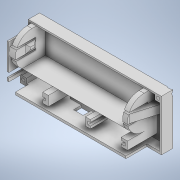
# Autodesk Inventor part: batteryholder18650
Saved by Autodesk Inventor 2022 (Build 260153000, 153)
## iProperties
Created: 2021-01-11
Part Number: batteryholder18650
Material: Generic
Document SubType Name: Modeling
Designer: papa
Density: 1 g/cm^3
Appearance: Default
Author: papa
Autodesk Inventor part; units mm, degrees
ref_plane "YZ Plane" through (0, 0, 0) normal (1, 0, 0) x (0, 1, 0)
ref_plane "XZ Plane" through (0, 0, 0) normal (0, 1, 0) x (-1, 0, 0)
ref_plane "XY Plane" through (0, 0, 0) normal (0, 0, 1) x (1, 0, 0)
sketch "Sketch1" plane through (0, 0, 0) normal (0, 0, 1) x (1, 0, 0)
  line L0 (0, 0) -> (82.5, 0)
  line L1 (82.5, 0) -> (82.5, 31.5)
  line L2 (82.5, 31.5) -> (0, 31.5)
  line L3 (0, 31.5) -> (0, 0)
  line L4 (1, 30.5) -> (81.5, 30.5)
  line L5 (81.5, 30.5) -> (81.5, 1.5)
  line L6 (81.5, 1.5) -> (1, 1.5)
  line L7 (1, 1.5) -> (1, 30.5)
  line L8 (81.5, 30.5) -> (78.5, 30.5)
  line L9 (78.5, 30.5) -> (78.5, 27.5)
  line L10 (78.5, 27.5) -> (81.5, 27.5)
  line L11 (81.5, 27.5) -> (81.5, 30.5)
  line L12 (1, 1.5) -> (4, 1.5)
  line L13 (4, 1.5) -> (4, 4.5)
  line L14 (4, 4.5) -> (1, 4.5)
  line L15 (1, 4.5) -> (1, 1.5)
  point P0 (78.5, 30.5)
  point P1 (1, 4.5)
  dimension "d0" = 82.5
  dimension "d1" = 31.5
  dimension "d2" = 1
  dimension "d3" = 1
  dimension "d4" = 1.5
  dimension "d5" = 1
  dimension "d26" = 4
  dimension "d27" = 4.5
  dimension "d28" = 4
  dimension "d29" = 4
  constraints: 32 end point, 8 parallel, 4 horizontal, 4 perpendicular
  measures "d0" distance of L2.end L1.end
  measures "d1" distance of L1.end L0.end
  measures "d2" distance between parallel lines of L4 L2
  measures "d3" distance between parallel lines of L3 L7
  measures "d4" distance between parallel lines of L0 L6
  measures "d5" distance between parallel lines of L1 L5
  measures "d26" distance between parallel lines of L3 L13
  measures "d27" distance between parallel lines of L0 L14
  measures "d28" distance between parallel lines of L2 L10
  measures "d29" distance between parallel lines of L1 L9
extrude "Extrusion1" add sketch "Sketch1" along normal blind 1.5 contours L3 L2 L1 L0 | L4 L9 L10 L5 L6 L13 L14 L7 | L4 L5 L10 L9 | L14 L13 L6 L7
extrude "Extrusion2" add sketch "Sketch1" along normal blind 20 contours L3 L2 L1 L0 | L4 L5 L10 L9 | L14 L13 L6 L7
sketch "Sketch2" plane through (0, 0, 0) normal (0, 0, -1) x (-1, 0, 0)
  circle A0 centre (-2, 2.5) radius 1
  circle A1 centre (-80.5, 29.5) radius 1
  line L0 (0, 0) -> (-82.5, 0) projected
  line L1 (0, 31.5) -> (0, 0) projected
  line L2 (-82.5, 0) -> (-82.5, 31.5) projected
  line L3 (-82.5, 31.5) -> (0, 31.5) projected
  dimension "d10" = 2
  dimension "d11" = 2
  dimension "d12" = 2.5
  dimension "d13" = 2
  dimension "d14" = 2
  dimension "d15" = 2
  constraints: 2 centre point
  measures "d10" diameter of A0
  measures "d11" diameter of A1
  measures "d12" distance from line of L0 A0.centre
  measures "d13" distance from line of L1 A0.centre
  measures "d14" distance from line of L2 A1.centre
  measures "d15" distance from line of L3 A1.centre
extrude "Extrusion3" cut sketch "Sketch2" against normal through all contours A0 | A1
sketch "Sketch3" plane through (0, 0, 20) normal (0, 0, 1) x (1, 0, 0)
  line L0 (82.5, 0) -> (82.5, 31.5) projected
  line L1 (0, 31.5) -> (82.5, 31.5)
  line L2 (82.5, 31.5) -> (82.5, 26.5)
  line L3 (82.5, 26.5) -> (0, 26.5)
  line L4 (0, 26.5) -> (0, 31.5)
  line L5 (0, 0) -> (5, 0)
  line L6 (5, 0) -> (5, 5)
  line L7 (5, 5) -> (0, 5)
  line L8 (0, 5) -> (0, 0)
  line L9 (82.5, 31.5) -> (0, 31.5) projected
  line L10 (82.5, 0) -> (73.5, 0)
  line L11 (73.5, 0) -> (73.5, 26.5)
  line L12 (73.5, 26.5) -> (82.5, 26.5)
  line L13 (82.5, 26.5) -> (82.5, 0)
  point P0 (1, 1.5)
  dimension "d20" = 5
  dimension "d21" = 5
  dimension "d22" = 5
  dimension "d125" = 9
  constraints: 24 end point, 6 parallel, 3 collinear, 3 horizontal, 3 perpendicular, 1 point on line
  measures "d20" distance between parallel lines of L1 L3
  measures "d21" distance between parallel lines of L8 L6
  measures "d22" distance of L7.end L5.start
  measures "d125" distance between parallel lines of L0 L11
extrude "Extrusion4" cut sketch "Sketch3" against normal blind 8
thicken "Thicken1" operation add thickness 5 both sides no extend neighbours yes toward (0, 0, -1) faces at (27.8333, 31.1667, 12)
sketch "Sketch4" plane through (0, 0, 1.5) normal (0, 0, 1) x (1, 0, 0)
  line L0 (74.5, 12) -> (74.5, 17.75)
  line L1 (74.5, 17.75) -> (71.5, 17.75)
  line L2 (71.5, 17.75) -> (71.5, 12)
  line L3 (71.5, 18.75) -> (74.5, 18.75)
  line L4 (74.5, 18.75) -> (74.5, 23.75)
  line L5 (74.5, 23.75) -> (71.5, 23.75)
  line L6 (71.5, 23.75) -> (71.5, 18.75)
  line L7 (78.5, 30.5) -> (1, 30.5) projected
  line L8 (71.5, 24.75) -> (74.5, 24.75)
  line L9 (74.5, 24.75) -> (74.5, 30.5)
  line L10 (74.5, 30.5) -> (71.5, 30.5)
  line L11 (71.5, 30.5) -> (71.5, 24.75)
  line L12 (5, 30.5) -> (2, 30.5)
  line L13 (2, 30.5) -> (2, 24.75)
  line L14 (2, 24.75) -> (5, 24.75)
  line L15 (5, 24.75) -> (5, 30.5)
  line L16 (5, 23.75) -> (1, 23.75)
  line L17 (1, 23.75) -> (1, 20)
  line L18 (1, 18.75) -> (5, 18.75)
  line L19 (5, 18.75) -> (5, 23.75)
  line L20 (5, 17.75) -> (2, 17.75)
  line L21 (2, 17.75) -> (2, 11.871)
  line L22 (5, 12) -> (5, 17.75)
  line L23 (71.5, 12) -> (5, 12)
  line L24 (2, 12) -> (2, 10)
  line L25 (2, 10) -> (74.5, 10)
  line L26 (74.5, 10) -> (74.5, 12)
  line L27 (1, 5) -> (1, 26.5) projected
  point P0 (0, 0)
  point P1 (2, 30.5)
  dimension "d31" = 1
  dimension "d32" = 1
  dimension "d33" = 3
  dimension "d35" = 3
  dimension "d76" = 66.5
  dimension "d80" = 18.5
  dimension "d126" = 1
  constraints: 52 end point, 11 parallel, 9 collinear, 9 point on line, 6 horizontal, 6 perpendicular
  measures "d31" distance between parallel lines of L5 L8
  measures "d32" distance between parallel lines of L1 L3
  measures "d33" distance between parallel lines of L13 L15
  measures "d35" distance between parallel lines of L2 L0
  measures "d76" distance between parallel lines of L19 L6
  measures "d80" distance between parallel lines of L7 L23
  measures "d126" distance between parallel lines of L27 L21
extrude "Extrusion5" add sketch "Sketch4" along normal up to surface (18.5 mm away)
chamfer "Chamfer3" distance 5 distance2 17 1 edges at (74.5, 21.25, 1.5) measured on face at (75, 21.25, 1.5)
sketch "Sketch9" plane through (74.5, 24.75, 1.5) normal (1, 0, 0) x (0, 0, -1)
  circle A0 centre (-8.25, -4.5) radius 10.25
  line L0 (-18.5, -1) -> (-18.5, -6) projected
  line L1 (0, -1) -> (-17, -1) projected
  line L2 (0, -14.75) -> (-18.5, -14.75) projected
  line L3 (-18.5, 5.75) -> (-18.5, 0) projected
  line L4 (-8.25, -14.75) -> (-18.5, -14.75)
  line L5 (-18.5, -14.75) -> (-18.5, 5.75)
  line L6 (-18.5, 5.75) -> (-8.25, 5.75)
  line L7 (-8.25, 5.75) -> (-8.25, -14.75)
  point P0 (1.5, -24.75)
  point P1 (-8.25, 5.75)
  point P2 (-18.5, -4.5)
  dimension "d73" = 20.5
  dimension "d72" = 10.25
  constraints: 8 end point, 2 parallel, 1 horizontal, 1 perpendicular, 1 point on line, 1 vertical, 3 other
  measures "d72" distance from line of L2 point (-8.25, -4.5)
extrude "Extrusion9" cut sketch "Sketch9" against normal up to surface (73.5 mm away) contours A0 L0 L5 L3 L6 | L2 L5 L0 A0
sketch "Sketch10" plane through (0, 0, 1.5) normal (0, 0, 1) x (1, 0, 0)
  line L0 (2, 10) -> (74.5, 10) projected
  line L1 (22, 10) -> (25.5, 10)
  line L2 (25.5, 10) -> (25.5, 4)
  line L3 (25.5, 4) -> (22, 4)
  line L4 (22, 7.5) -> (23.5, 7.5)
  line L5 (23.5, 7.5) -> (23.5, 6)
  line L6 (23.5, 6) -> (22, 6)
  line L7 (22, 4) -> (22, 6)
  line L8 (22, 7.5) -> (22, 10)
  line L9 (1, 5) -> (1, 20.25) projected
  point P0 (0, 0)
  dimension "d81" = 2
  dimension "d82" = 2
  dimension "d83" = 22.5
  dimension "d84" = 1.5
  dimension "d85" = 2.5
  dimension "d86" = 1.5
  constraints: 16 end point, 4 parallel, 2 horizontal, 2 perpendicular, 1 collinear, 1 point on line
  measures "d81" distance between parallel lines of L3 L6
  measures "d82" distance between parallel lines of L2 L5
  measures "d83" distance between parallel lines of L5 L9
  measures "d84" distance between parallel lines of L5 L7
  measures "d85" distance between parallel lines of L0 L4
  measures "d86" distance between parallel lines of L6 L4
extrude "Extrusion10" add sketch "Sketch10" along normal up to surface (18.5 mm away)
sketch "Sketch11" plane through (1, 4.5, 12) normal (1, 0, 0) x (0, 0, -1)
  line L0 (6, 5.5) -> (-8, 5.5)
  line L1 (-8, 5.5) -> (-8, 2.5)
  line L2 (-8, 2.5) -> (6, 2.5)
  line L3 (6, 2.5) -> (6, 5.5)
  line L4 (12, 27) -> (12, -4.5) projected
  line L5 (10.5, 14.25) -> (10.5, 0) projected
  dimension "d94" = 3
  dimension "d128" = 4.5
  constraints: 8 end point, 2 parallel, 1 horizontal, 1 perpendicular
  measures "d94" distance between parallel lines of L2 L0
  measures "d128" distance between parallel lines of L5 L3
extrude "Extrusion11" cut sketch "Sketch11" against normal through all
sketch "Sketch12" plane through (0, 0, 1.5) normal (0, 0, 1) x (1, 0, 0)
  line L0 (25.5, 10) -> (74.5, 10) projected
  line L1 (51.5, 10) -> (48.5, 10)
  line L2 (48.5, 10) -> (48.5, 5)
  line L3 (48.5, 5) -> (51.5, 5)
  line L4 (74.5, 10) -> (70.5, 10)
  line L5 (70.5, 5) -> (74.5, 5)
  line L6 (74.5, 5) -> (74.5, 10)
  line L7 (51.5, 8.5) -> (50, 8.5)
  line L8 (50, 8.5) -> (50, 6.5)
  line L9 (50, 6.5) -> (51.5, 6.5)
  line L10 (70.5, 8.5) -> (73, 8.5)
  line L11 (73, 8.5) -> (73, 6.5)
  line L12 (73, 6.5) -> (70.5, 6.5)
  line L13 (51.5, 5) -> (51.5, 6.5)
  line L14 (51.5, 8.5) -> (51.5, 10)
  line L15 (70.5, 10) -> (70.5, 8.5)
  line L16 (70.5, 6.5) -> (70.5, 5)
  point P0 (0, 0)
  dimension "d97" = 1.5
  dimension "d98" = 1.5
  dimension "d99" = 1.5
  dimension "d100" = 23
  dimension "d141" = 2
  dimension "d142" = 5
  dimension "d143" = 3
  constraints: 32 end point, 8 parallel, 5 perpendicular, 4 horizontal, 4 point on line, 2 collinear
  measures "d97" distance of L4.end L10.start
  measures "d98" distance between parallel lines of L6 L11
  measures "d99" distance between parallel lines of L2 L8
  measures "d100" distance between parallel lines of L11 L8
  measures "d141" distance between parallel lines of L9 L7
  measures "d142" distance between parallel lines of L3 L0
  measures "d143" distance of L2.end L3.end
extrude "Extrusion12" add sketch "Sketch12" along normal up to surface (18.5 mm away)
sketch "Sketch13" plane through (0, 0, 1.5) normal (0, 0, 1) x (1, 0, 0)
  line L0 (4, 1.5) -> (81.5, 1.5) projected
  line L1 (25.5, 1.5) -> (45.5, 1.5)
  line L2 (45.5, 1.5) -> (45.5, 6.5)
  line L3 (45.5, 6.5) -> (25.5, 6.5)
  line L4 (25.5, 6.5) -> (25.5, 1.5)
  line L5 (25.5, 10) -> (25.5, 4) projected
  circle A0 centre (28, 4) radius 1.75
  circle A1 centre (43, 4) radius 1.75
  point P0 (0, 0)
  point P1 (45.5, 1.5)
  dimension "d106" = 20
  dimension "d107" = 3.5
  dimension "d108" = 3.5
  dimension "d110" = 2.5
  dimension "d111" = 2.5
  dimension "d112" = 2.5
  dimension "d113" = 2.5
  dimension "d114" = 5
  constraints: 8 end point, 2 centre point, 2 parallel, 1 collinear, 1 horizontal, 1 perpendicular, 1 point on line
  measures "d106" distance of L2.end L3.end
  measures "d107" diameter of A0
  measures "d108" diameter of A1
  measures "d110" distance from line of L4 A0.centre
  measures "d111" distance from line of L2 A1.centre
  measures "d112" distance from line of L3 A0.centre
  measures "d113" distance from line of L3 A1.centre
  measures "d114" distance between parallel lines of L0 L3
extrude "Extrusion13" add sketch "Sketch13" along normal blind 5
sketch "Sketch14" plane through (5, 1.5, 20) normal (0, 1, 0) x (1, 0, 0)
  line L0 (40.5, 13.5) -> (20.5, 13.5) projected
  line L1 (27.5, 13.5) -> (33.5, 13.5)
  line L2 (33.5, 13.5) -> (33.5, 8.5)
  line L3 (33.5, 8.5) -> (27.5, 8.5)
  line L4 (27.5, 8.5) -> (27.5, 13.5)
  line L5 (20.5, 10.25) -> (20.5, 18.5) projected
  point P0 (-5, 20)
  dimension "d117" = 6
  dimension "d118" = 5
  dimension "d119" = 7
  constraints: 8 end point, 2 parallel, 1 horizontal, 1 perpendicular, 1 point on line
  measures "d117" distance between parallel lines of L2 L4
  measures "d118" distance between parallel lines of L0 L3
  measures "d119" distance between parallel lines of L5 L4
extrude "Extrusion14" cut sketch "Sketch14" against normal through all
sketch "Sketch15" plane through (0, 0, 1.5) normal (0, 0, 1) x (1, 0, 0)
  line L0 (5, 24.75) -> (2, 24.75) projected
  line L1 (1, 23.75) -> (5, 23.75) projected
  line L2 (2, 24.75) -> (5, 24.75)
  line L3 (5, 24.75) -> (5, 23.75)
  line L4 (5, 23.75) -> (2, 23.75)
  line L5 (2, 23.75) -> (2, 24.75)
  line L6 (2, 17.75) -> (5, 17.75) projected
  line L7 (5, 18.75) -> (1, 18.75) projected
  line L8 (2, 17.75) -> (5, 17.75)
  line L9 (5, 17.75) -> (5, 18.75)
  line L10 (5, 18.75) -> (2, 18.75)
  line L11 (2, 18.75) -> (2, 17.75)
  line L12 (74.5, 18.75) -> (71.5, 18.75) projected
  line L13 (74.5, 10) -> (74.5, 17.75) projected
  line L14 (71.5, 18.75) -> (74.5, 18.75)
  line L15 (74.5, 18.75) -> (74.5, 17.75)
  line L16 (74.5, 17.75) -> (71.5, 17.75)
  line L17 (71.5, 17.75) -> (71.5, 18.75)
  line L18 (74.5, 24.75) -> (74.5, 30.5) projected
  line L19 (71.5, 23.75) -> (74.5, 23.75) projected
  line L20 (74.5, 24.75) -> (71.5, 24.75)
  line L21 (71.5, 24.75) -> (71.5, 23.75)
  line L22 (71.5, 23.75) -> (74.5, 23.75)
  line L23 (74.5, 23.75) -> (74.5, 24.75)
  point P0 (0, 0)
  constraints: 32 end point, 8 parallel, 4 horizontal, 4 perpendicular
extrude "Extrusion15" add sketch "Sketch15" along normal blind 6
sketch "Sketch16" plane through (5, 12, 1.5) normal (1, 0, 0) x (0, 0, -1)
  line L0 (-6, 12.75) -> (-6, 11.75) projected
  line L1 (-6, 11.75) -> (-12, 11.75)
  line L2 (-12, 11.75) -> (-12, 6.75)
  line L3 (-12, 6.75) -> (-6, 6.75)
  line L4 (-6, 6.75) -> (-6, 11.75)
  point P0 (1.5, -12)
  dimension "d131" = 6
  dimension "d132" = 5
  constraints: 8 end point, 2 parallel, 1 horizontal, 1 perpendicular
  measures "d131" distance of L3.end L2.end
  measures "d132" distance of L2.end L1.end
extrude "Extrusion16" add sketch "Sketch16" along normal blind 1 draft -60
sketch "Sketch17" plane through (71.5, 12, 1.5) normal (-1, 0, 0) x (0, 0, 1)
  line L0 (6, 11.75) -> (0, 11.75) projected
  line L1 (0, 6.75) -> (18.3896, 6.75) projected
  line L2 (6, 11.75) -> (12, 11.75)
  line L3 (12, 11.75) -> (12, 6.75)
  line L4 (12, 6.75) -> (6, 6.75)
  line L5 (6, 6.75) -> (6, 11.75)
  point P0 (-1.5, -12)
  point P1 (6, 6.75)
  dimension "d135" = 6
  constraints: 8 end point, 2 parallel, 1 horizontal, 1 perpendicular, 1 point on line
  measures "d135" distance of L3.end L4.end
extrude "Extrusion17" add sketch "Sketch17" along normal blind 1 draft -60
chamfer "Chamfer7" distance 1.5 angle 45 2 edges at (3, 2.5, 0) (81.5, 29.5, 0)
equation "\"d98\" = d97"
equation "\"d99\" = d97"
body "Solid1"
